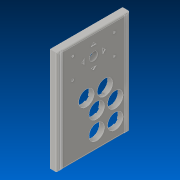
# Autodesk Inventor part: Top
Saved by Autodesk Inventor 2016 (Build 200138000, 138)
## iProperties
Created: 2015-08-21
Part Number: Top
Material: Generic
Document SubType Name: Modeling
Designer: Moffitt
Density: 1 g/cm^3
Appearance: Default
Author: Moffitt
Autodesk Inventor part; units mm, degrees
ref_plane "YZ Plane" through (0, 0, 0) normal (1, 0, 0) x (0, 1, 0)
ref_plane "XZ Plane" through (0, 0, 0) normal (0, 1, 0) x (-1, 0, 0)
ref_plane "XY Plane" through (0, 0, 0) normal (0, 0, 1) x (1, 0, 0)
sketch "Top-Body" plane through (0, 0, 0) normal (1, 0, 0) x (0, 1, 0)
  line L0 (107.2007, 64.0864) -> (-92.7993, 64.0864)
  line L1 (-92.7993, 64.0864) -> (-92.7993, -75.9136)
  line L2 (-92.7993, -75.9136) -> (107.2007, -75.9136)
  line L3 (107.2007, -75.9136) -> (107.2007, 64.0864)
  circle A0 centre (67.2007, -5.9136) radius 8
  circle A1 centre (4.2007, -27.9136) radius 15
  circle A2 centre (-26.2993, -47.9136) radius 15
  circle A3 centre (-62.2993, -47.9136) radius 15
  circle A4 centre (4.2007, 8.0864) radius 15
  circle A5 centre (-26.2993, -11.9136) radius 15
  circle A6 centre (-62.2993, -11.9136) radius 15
  circle A7 centre (87.2007, 34.0864) radius 2
  circle A8 centre (87.2007, -45.9136) radius 2.0363
  circle A9 centre (47.2007, -45.9136) radius 1.917
  circle A10 centre (47.2007, 34.619) radius 2.4037
  point P0 (0, 0)
  dimension "d0" = 200
  dimension "d1" = 140
  dimension "d2" = 16
  dimension "d3" = 40
  dimension "d5" = 30
  dimension "d6" = 30
  dimension "d7" = 20
  dimension "d8" = 30.5
  dimension "d9" = 30
  dimension "d10" = 36
  dimension "d11" = 0
  dimension "d12" = 63
  dimension "d13" = 30
  dimension "d14" = 30
  dimension "d15" = 30
  dimension "d16" = 36
  dimension "d17" = 36
  dimension "d18" = 36
  dimension "d19" = 0
  dimension "d20" = 0
  dimension "d21" = 0
  dimension "d23" = 14
  dimension "d24" = 70
  dimension "d25" = 4
  dimension "d26" = 40
  dimension "d27" = 20
  dimension "d28" = 20
  dimension "d29" = 20
  dimension "d30" = 20
  dimension "d31" = 40
  dimension "d32" = 40
  dimension "d33" = 70
  constraints: 11 centre point, 8 end point, 2 parallel, 1 horizontal, 1 perpendicular
  measures "d0" distance of L0.start L0.end
  measures "d1" distance of L2.end L0.start
  measures "d2" diameter of A0
  measures "d3" distance from line of L3 A0.centre
  measures "d5" diameter of A1
  measures "d6" diameter of A2
  measures "d7" vertical distance of A2.centre A1.centre
  measures "d8" horizontal distance of A2.centre A1.centre
  measures "d9" diameter of A3
  measures "d10" distance of A3.centre A2.centre
  measures "d11" vertical distance of A3.centre A2.centre
  measures "d12" horizontal distance of A1.centre A0.centre
  measures "d13" diameter of A4
  measures "d14" diameter of A5
  measures "d15" diameter of A6
  measures "d16" distance of A1.centre A4.centre
  measures "d17" distance of A2.centre A5.centre
  measures "d18" distance of A3.centre A6.centre
  measures "d19" horizontal distance of A4.centre A1.centre
  measures "d20" horizontal distance of A5.centre A2.centre
  measures "d21" horizontal distance of A6.centre A3.centre
  measures "d23" vertical distance of A0.centre A4.centre
  measures "d24" distance from line of L2 A0.centre
  measures "d25" diameter of A7
  measures "d26" vertical distance of A0.centre A7.centre
  measures "d27" horizontal distance of A7.centre A0.centre
  measures "d28" horizontal distance of A10.centre A0.centre
  measures "d29" horizontal distance of A0.centre A8.centre
  measures "d30" horizontal distance of A9.centre A0.centre
  measures "d31" vertical distance of A0.centre A8.centre
  measures "d32" vertical distance of A9.centre A0.centre
  measures "d33" distance from line of L0 A0.centre
extrude "Main Face" add sketch "Top-Body" along normal blind 10
fillet "Top Fillet" radius 3 4 edges at (10, 107.2007, -5.9136) (10, 7.2007, 64.0864) (10, 7.2007, -75.9136) (10, -92.7993, -5.9136)
sketch "Button clip cutouts" plane through (0, 0, 0) normal (-1, 0, 0) x (0, 0, 1)
  line L0 (-33.0644, -53.1069) -> (-38.7212, -47.45)
  line L1 (-38.7212, -47.45) -> (-62.7628, -71.4917)
  line L2 (-62.7628, -71.4917) -> (-57.106, -77.1485)
  line L3 (-57.106, -77.1485) -> (-33.0644, -53.1069)
  line L4 (64.0864, -92.7993) -> (-75.9136, -92.7993) projected
  line L5 (2.9356, -71.4917) -> (-2.7212, -77.1485)
  line L6 (-2.7212, -77.1485) -> (-26.7628, -53.1069)
  line L7 (-26.7628, -53.1069) -> (-21.106, -47.45)
  line L8 (-21.106, -47.45) -> (2.9356, -71.4917)
  line L9 (-21.106, -41.1485) -> (-26.7628, -35.4917)
  line L10 (-26.7628, -35.4917) -> (-2.7212, -11.45)
  line L11 (-2.7212, -11.45) -> (2.9356, -17.1069)
  line L12 (2.9356, -17.1069) -> (-21.106, -41.1485)
  line L13 (-38.7212, -41.1485) -> (-33.0644, -35.4917)
  line L14 (-33.0644, -35.4917) -> (-57.106, -11.45)
  line L15 (-57.106, -11.45) -> (-62.7628, -17.1069)
  line L16 (-62.7628, -17.1069) -> (-38.7212, -41.1485)
  circle A0 centre (-47.9136, -26.2993) radius 15 projected
  circle A1 centre (-11.9136, -26.2993) radius 15 projected
  line L17 (-1.106, -10.6485) -> (-6.7628, -4.9917)
  line L18 (-6.7628, -4.9917) -> (17.2788, 19.05)
  line L19 (17.2788, 19.05) -> (22.9356, 13.3931)
  line L20 (22.9356, 13.3931) -> (-1.106, -10.6485)
  line L21 (-23.9136, -12.7993) -> (-31.9136, -12.7993)
  line L22 (-31.9136, -12.7993) -> (-31.9136, 21.2007)
  line L23 (-31.9136, 21.2007) -> (-23.9136, 21.2007)
  line L24 (-23.9136, 21.2007) -> (-23.9136, -12.7993)
  circle A2 centre (8.0864, 4.2007) radius 15 projected
  circle A3 centre (-27.9136, 4.2007) radius 15 projected
  point P0 (0, 0)
  point P1 (-11.9136, -62.2993)
  point P2 (-47.9136, -62.2993)
  dimension "d46" = 45
  dimension "d48" = 17
  dimension "d49" = 4
  dimension "d50" = 4
  dimension "d52" = 4
  dimension "d53" = 4
  dimension "d54" = 17
  dimension "d55" = 17
  dimension "d56" = 17
  dimension "d57" = 90
  dimension "d58" = 90
  dimension "d59" = 90
  dimension "d60" = 90
  dimension "d61" = 90
  dimension "d62" = 90
  dimension "d63" = 34
  dimension "d64" = 8
  dimension "d65" = 8
  dimension "d66" = 4
  dimension "d67" = 17
  dimension "d68" = 34
  dimension "d69" = 8
  dimension "d70" = 90
  dimension "d73" = 17
  dimension "d74" = 4
  dimension "d77" = 135
  dimension "d78" = 90
  dimension "d79" = 90
  dimension "d81" = 90
  dimension "d82" = 90
  dimension "d83" = 90
  dimension "d85" = 90
  dimension "d86" = 90
  dimension "d87" = 90
  dimension "d88" = 34
  dimension "d89" = 8
  dimension "d90" = 4
  dimension "d91" = 17
  dimension "d92" = 90
  dimension "d93" = 90
  dimension "d94" = 34
  dimension "d95" = 17
  dimension "d96" = 4
  dimension "d97" = 8
  constraints: 48 end point, 10 perpendicular, 1 horizontal, 1 parallel, 1 point on line
  measures "d46" angle of L4 L3
  measures "d48" distance from line of L0 point (-47.914, -62.299)
  measures "d49" distance from line of L1 point (-47.914, -62.299)
  measures "d50" distance from line of L3 point (-47.914, -62.299)
  measures "d52" distance from line of L8 point (-11.914, -62.299)
  measures "d53" distance from line of L6 point (-11.914, -62.299)
  measures "d54" distance from line of L5 point (-11.914, -62.299)
  measures "d55" distance from line of L7 point (-11.914, -62.299)
  measures "d56" distance from line of L2 point (-47.914, -62.299)
  measures "d57" angle of L10 L9
  measures "d58" angle of L11 L12
  measures "d59" angle of L9 L12
  measures "d60" angle of L10 L11
  measures "d61" angle of L16 L13
  measures "d62" angle of L15 L14
  measures "d63" distance between parallel lines of L15 L13
  measures "d64" distance of L13.start L13.end
  measures "d65" distance of L14.end L15.end
  measures "d66" distance from line of L14 A0.centre
  measures "d67" distance from line of L13 A0.centre
  measures "d68" distance of L9.end L10.end
  measures "d69" distance of L9.start L9.end
  measures "d70" angle of L14 L10
  measures "d73" distance from line of A1.centre L11
  measures "d74" distance from line of L10 A1.centre
  measures "d77" angle of L4 L8
  measures "d78" angle of L5 L8
  measures "d79" angle of L6 L7
  measures "d81" angle of L8 L12
  measures "d82" angle of L6 L3
  measures "d83" angle of L16 L1
  measures "d85" angle of L17 L20
  measures "d86" angle of L20 L19
  measures "d87" angle of L17 L10
  measures "d88" distance of L19.end L17.start
  measures "d89" distance of L18.end L19.end
  measures "d90" distance from line of L20 A2.centre
  measures "d91" distance from line of L17 A2.centre
  measures "d92" angle of L21 L24
  measures "d93" angle of L23 L22
  measures "d94" distance of L21.end L22.end
  measures "d95" distance from line of L21 A3.centre
  measures "d96" distance from line of L22 A3.centre
  measures "d97" distance of L22.end L23.end
extrude "Button Snap Cutouts" cut sketch "Button clip cutouts" against normal blind 7 contours L3 L2 L1 L0 | L5 L6 L7 L8 | L9 L10 A1 L12 | A1 L10 L12 | A1 L10 L11 L12 | L16 A0 L14 L13 | L16 A0 L14 | L16 L15 L14 A0 | L17 L18 A2 L20 | A2 L18 L20 | A2 L18 L19 L20 | L21 L22 A3 L24 | A3 L22 L24 | A3 L22 L23 L24
chamfer "Button Snap Chamfers" distance 0.5 angle 45 48 edges at (3.5, -69.6934, -60.9645) (3.5, -49.2483, -40.5195) (3.5, -54.9052, -34.8626) (3.5, -54.9052, -24.9645) (3.5, -49.2483, -19.3077) (3.5, -75.3502, -4.5195) (3.5, -69.6934, 1.1374) (3.5, -75.3502, -55.3077) (3.5, -77.1485, -57.106) (3.5, -71.4917, -62.7628) (3.5, -47.45, -38.7212) (3.5, -53.1069, -33.0644) (3.5, -53.1069, -26.7628) (3.5, -47.45, -21.106) (3.5, -71.4917, 2.9356) (3.5, -77.1485, -2.7212) (3.5, -39.3502, -40.5195) (3.5, -41.1485, -38.7212) (3.5, -35.4917, -33.0644) (3.5, -33.6934, -34.8626) (3.5, -13.2483, -55.3077) (3.5, -11.45, -57.106) (3.5, -18.9052, -60.9645) (3.5, -17.1069, -62.7628) (3.5, -35.4917, -26.7628) (3.5, -41.1485, -21.106) (3.5, -39.3502, -19.3077) (3.5, -33.6934, -24.9645) (3.5, -13.2483, -4.5195) (3.5, -11.45, -2.7212) (3.5, -17.1069, 2.9356) (3.5, -18.9052, 1.1374) (3.5, -10.2561, -23.9136) (3.5, -12.7993, -23.9136) (3.5, -12.7993, -31.9136) (3.5, -10.2561, -31.9136) (3.5, 18.6576, -31.9136) (3.5, 21.2007, -31.9136) (3.5, 21.2007, -23.9136) (3.5, 18.6576, -23.9136) (3.5, -3.1934, -4.9645) (3.5, -4.9917, -6.7628) (3.5, -10.6485, -1.106) (3.5, -8.8502, 0.6923) (3.5, 17.2517, 15.4805) (3.5, 19.05, 17.2788) (3.5, 13.3931, 22.9356) (3.5, 11.5948, 21.1374)
sketch "sweet lines" plane through (0, -92.7993, -75.9136) normal (0, -1, 0) x (1, 0, 0)
  line L0 (10, 137) -> (10, 3) projected
  line L1 (10, 4.5) -> (8.5, 4.5)
  line L2 (8.5, 4.5) -> (8.5, 6.5)
  line L3 (8.5, 6.5) -> (10, 6.5)
  line L4 (10, 6.5) -> (10, 4.5)
  line L5 (10, 8.5) -> (8.5, 8.5)
  line L6 (8.5, 8.5) -> (8.5, 10.5)
  line L7 (8.5, 10.5) -> (10, 10.5)
  line L8 (10, 10.5) -> (10, 8.5)
  line L9 (10, 135.5) -> (8.5, 135.5)
  line L10 (8.5, 135.5) -> (8.5, 133.5)
  line L11 (8.5, 133.5) -> (10, 133.5)
  line L12 (10, 133.5) -> (10, 135.5)
  line L13 (10, 132) -> (8.5, 132)
  line L14 (8.5, 132) -> (8.5, 130)
  line L15 (8.5, 130) -> (10, 130)
  line L16 (10, 130) -> (10, 132)
  point P0 (0, 75.9136)
  dimension "d103" = 2
  dimension "d104" = 1.5
  dimension "d105" = 2
  dimension "d106" = 2
  dimension "d107" = 1.5
  dimension "d110" = 1.5
  dimension "d111" = 2
  dimension "d112" = 2
  dimension "d113" = 1.5
  dimension "d114" = 1.5
  dimension "d115" = 1.5
  dimension "d116" = 1.5
  constraints: 32 end point, 8 parallel, 5 point on line, 4 horizontal, 4 perpendicular
  measures "d103" distance of L1.end L2.end
  measures "d104" distance of L1.start L1.end
  measures "d105" distance between parallel lines of L5 L3
  measures "d106" distance of L5.end L6.end
  measures "d107" distance of L5.start L5.end
  measures "d110" distance from line of L0.end L1
  measures "d111" distance of L13.end L14.end
  measures "d112" distance of L9.end L10.end
  measures "d113" distance from line of L9 L0.start
  measures "d114" distance between parallel lines of L13 L11
  measures "d115" distance of L14.end L15.end
  measures "d116" distance of L10.end L11.end
extrude "SNOW WHITE DESIGN PATTERNS" cut sketch "sweet lines" against normal blind 200
sketch "Insignias" plane through (10, 0, 0) normal (1, 0, 0) x (0, 0, -1)
  line L0 (23.9136, 72.2007) -> (23.9136, 62.2007)
  line L1 (23.9136, 62.2007) -> (28.9136, 67.2007)
  line L2 (28.9136, 67.2007) -> (23.9136, 72.2007)
  circle A0 centre (5.9136, 67.2007) radius 8 projected
  line L3 (10.9136, 49.2007) -> (0.9136, 49.2007)
  line L4 (0.9136, 49.2007) -> (5.9136, 44.2007)
  line L5 (5.9136, 44.2007) -> (10.9136, 49.2007)
  line L6 (10.9136, 85.2007) -> (0.9136, 85.2007)
  line L7 (0.9136, 85.2007) -> (5.9136, 90.2007)
  line L8 (5.9136, 90.2007) -> (10.9136, 85.2007)
  line L9 (-12.0864, 62.2007) -> (-12.0864, 72.2007)
  line L10 (-12.0864, 72.2007) -> (-17.0864, 67.2007)
  line L11 (-17.0864, 67.2007) -> (-12.0864, 62.2007)
  point P0 (0, 0)
  dimension "d117" = 45
  dimension "d118" = 45
  dimension "d119" = 10
  dimension "d120" = 10
  dimension "d121" = 5
  dimension "d122" = 45
  dimension "d123" = 45
  dimension "d124" = 10
  dimension "d125" = 10
  dimension "d126" = 5
  dimension "d127" = 18
  dimension "d128" = 18
  dimension "d129" = 18
  constraints: 24 end point, 3 perpendicular, 2 horizontal, 2 point on line, 1 vertical
  measures "d117" angle of L0 L2
  measures "d118" angle of L0 L1
  measures "d119" distance of L0.start L0.end
  measures "d120" distance edge to line of A0 L0
  measures "d121" vertical distance of A0.centre L0.start
  measures "d122" angle of L5 L3
  measures "d123" angle of L3 L4
  measures "d124" distance of L3.start L3.end
  measures "d125" distance edge to line of A0 L3
  measures "d126" horizontal distance of L3.end A0.centre
  measures "d127" distance from line of A0.centre L0
  measures "d128" distance from line of A0.centre L6
  measures "d129" distance from line of L9 A0.centre
extrude "Insignias Extrusion" cut sketch "Insignias" against normal blind 1.5 contours L2 L1 L0 | L5 L4 L3 | L6 L7 L8 | L11 L10 L9
sketch "Border" plane through (0, 0, 0) normal (-1, 0, 0) x (0, 0, 1)
  line L0 (-71.9136, -90.7993) -> (60.0864, -90.7993)
  line L1 (60.0864, -90.7993) -> (60.0864, 105.2007)
  line L2 (60.0864, 105.2007) -> (-71.9136, 105.2007)
  line L3 (-71.9136, 105.2007) -> (-71.9136, -90.7993)
  line L4 (64.0864, -92.7993) -> (-75.9136, -92.7993) projected
  line L5 (-75.9136, 107.2007) -> (64.0864, 107.2007) projected
  line L6 (-75.9136, -92.7993) -> (-75.9136, 107.2007) projected
  line L7 (64.0864, 107.2007) -> (64.0864, -92.7993) projected
  point P0 (0, 0)
  dimension "d132" = 2
  dimension "d133" = 2
  dimension "d134" = 4
  dimension "d135" = 4
  constraints: 8 end point, 2 parallel, 1 horizontal, 1 perpendicular
  measures "d132" distance between parallel lines of L4 L0
  measures "d133" distance between parallel lines of L5 L2
  measures "d134" distance between parallel lines of L6 L3
  measures "d135" distance between parallel lines of L7 L1
extrude "Connection Lip" add sketch "Border" along normal blind 4
body "Solid1"
